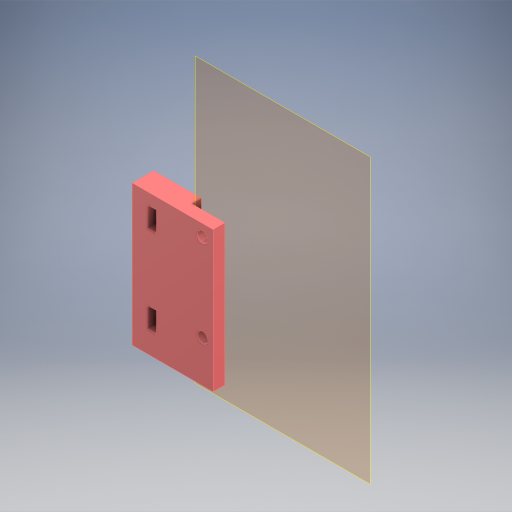
# Autodesk Inventor part: foot_right_connection
Saved by Autodesk Inventor 2024 (Build 280153000, 153)
## iProperties
Created: 2024-09-03
Part Number: foot_right_connection
Material: PMMA 플라스틱
Document SubType Name: Modeling
Designer: msi
Density: 1.188 g/cm^3
Appearance: 매끄러움 - 빨간색
Author: msi
Autodesk Inventor part; units mm, degrees
ref_plane "YZ Plane" through (0, 0, 0) normal (1, 0, 0) x (0, 1, 0)
ref_plane "XZ Plane" through (0, 0, 0) normal (0, 1, 0) x (-1, 0, 0)
ref_plane "XY Plane" through (0, 0, 0) normal (0, 0, 1) x (1, 0, 0)
ref_plane "작업 평면1" through (0, 0, 0) normal (0, 0, 1) x (1, 0, 0)
sketch "스케치2" plane through (0, 0, 0) normal (0, 0, 1) x (1, 0, 0)
  line L0 (13.5, -39.75) -> (11.5, -39.75) projected
  arc A0 (11.5, -39.75) -> (9.25, -42) centre (11.5, -42) ccw projected
  line L1 (9.25, -42) -> (9.25, -44) projected
  arc A1 (8.25, -45) -> (9.25, -44) centre (8.25, -44) ccw projected
  line L2 (8.25, -45) -> (-8.25, -45) projected
  arc A2 (-9.25, -44) -> (-8.25, -45) centre (-8.25, -44) ccw projected
  line L3 (-9.25, -44) -> (-9.25, -42) projected
  arc A3 (-9.25, -42) -> (-11.5, -39.75) centre (-11.5, -42) ccw projected
  line L4 (-11.5, -39.75) -> (-13.5, -39.75) projected
  arc A4 (-14.5, -38.75) -> (-13.5, -39.75) centre (-13.5, -38.75) ccw projected
  line L5 (-14.5, -38.75) -> (-14.5, 8.25) projected
  arc A5 (-13.5, 9.25) -> (-14.5, 8.25) centre (-13.5, 8.25) ccw projected
  line L6 (-13.5, 9.25) -> (-11.5, 9.25) projected
  arc A6 (-11.5, 9.25) -> (-9.25, 11.5) centre (-11.5, 11.5) ccw projected
  line L7 (-9.25, 11.5) -> (-9.25, 14.5) projected
  line L8 (-15, 14.5) -> (-9.25, 14.5) projected
  line L9 (-20.1, 8.5) -> (-15, 14.5) projected
  line L10 (-20.1, -44.6) -> (-20.1, 8.5) projected
  line L11 (-15, -50.6) -> (-20.1, -44.6) projected
  line L12 (15, -50.6) -> (-15, -50.6) projected
  line L13 (20.1, -44.6) -> (15, -50.6) projected
  line L14 (20.1, 8.5) -> (20.1, -44.6) projected
  line L15 (15, 14.5) -> (20.1, 8.5) projected
  line L16 (9.25, 14.5) -> (15, 14.5) projected
  line L17 (9.25, 14.5) -> (9.25, 11.5) projected
  arc A7 (9.25, 11.5) -> (11.5, 9.25) centre (11.5, 11.5) ccw projected
  line L18 (11.5, 9.25) -> (13.5, 9.25) projected
  arc A8 (14.5, 8.25) -> (13.5, 9.25) centre (13.5, 8.25) ccw projected
  line L19 (14.5, 8.25) -> (14.5, -38.75) projected
  arc A9 (13.5, -39.75) -> (14.5, -38.75) centre (13.5, -38.75) ccw projected
  circle A10 centre (17.3, 4) radius 1.35 projected
  circle A11 centre (17.3, -18) radius 1.35 projected
  circle A12 centre (11, -47.8) radius 1.35 projected
  circle A13 centre (-17.3, 4) radius 1.35 projected
  circle A14 centre (-17.3, -18) radius 1.35 projected
  circle A15 centre (-11, -47.8) radius 1.35 projected
  circle A16 centre (17.3, -40) radius 1.35 projected
  circle A17 centre (-17.3, -40) radius 1.35 projected
  line L20 (-43, 2.0766) -> (-43, -42.1766) projected
  line L21 (-14.6, 8.25) -> (-14.6, -38.75)
  arc A18 (-14.6, -38.75) -> (-13.5, -39.85) centre (-13.5, -38.75) ccw
  line L22 (-13.5, -39.85) -> (-11.5, -39.85)
  arc A19 (-9.35, -42) -> (-11.5, -39.85) centre (-11.5, -42) ccw
  line L23 (-9.35, -42) -> (-9.35, -44)
  arc A20 (-9.35, -44) -> (-8.25, -45.1) centre (-8.25, -44) ccw
  line L24 (-8.25, -45.1) -> (8.25, -45.1)
  arc A21 (8.25, -45.1) -> (9.35, -44) centre (8.25, -44) ccw
  line L25 (9.35, -44) -> (9.35, -42)
  arc A22 (11.5, -39.85) -> (9.35, -42) centre (11.5, -42) ccw
  line L26 (11.5, -39.85) -> (13.5, -39.85)
  arc A23 (13.5, -39.85) -> (14.6, -38.75) centre (13.5, -38.75) ccw
  line L27 (14.6, -38.75) -> (14.6, 8.25)
  arc A24 (14.6, 8.25) -> (13.5, 9.35) centre (13.5, 8.25) ccw
  line L28 (13.5, 9.35) -> (11.5, 9.35)
  arc A25 (9.35, 11.5) -> (11.5, 9.35) centre (11.5, 11.5) ccw
  line L29 (9.35, 11.5) -> (9.35, 14.4)
  line L30 (9.35, 14.4) -> (14.9538, 14.4)
  line L31 (14.9538, 14.4) -> (20, 8.4632)
  line L32 (20, 8.4632) -> (20, -44.5632)
  line L33 (20, -44.5632) -> (14.9538, -50.5)
  line L34 (14.9538, -50.5) -> (-14.9538, -50.5)
  line L35 (-20, -15) -> (-20, 8.4632)
  line L36 (-20, 8.4632) -> (-14.9538, 14.4)
  line L37 (-14.9538, 14.4) -> (-9.35, 14.4)
  line L38 (-9.35, 14.4) -> (-9.35, 11.5)
  arc A26 (-11.5, 9.35) -> (-9.35, 11.5) centre (-11.5, 11.5) ccw
  line L39 (-11.5, 9.35) -> (-13.5, 9.35)
  arc A27 (-13.5, 9.35) -> (-14.6, 8.25) centre (-13.5, 8.25) ccw
  line L40 (-20, -15) -> (-14.6, -15)
  line L41 (-14.6, -15) -> (-14.6, -45)
  line L42 (-43, -15) -> (-20, -15)
  line L43 (-35, -45) -> (-35, -50.5)
  line L44 (-35, -50.5) -> (-14.6, -50.5)
  line L45 (-14.6, -50.5) -> (-14.6, -45)
  line L46 (-35, -45) -> (-35, -15)
  point P0 (0, 0)
  point P1 (-14.6, -38.75)
  point P2 (-14.6, -50.5)
  point P3 (-14.6, -38.75)
  dimension "d1" = 0.1
  dimension "d27" = 20.4
  constraints: 52 end point, 20 point on circle, 10 centre point, 2 point on line, 1 parallel, 1 perpendicular, 26 other
  measures "d1" distance between parallel lines of L5 L21
  measures "d27" distance between parallel lines of L43 L45
extrude "돌출8" add sketch "스케치2" along normal blind 3 contours L44 L43 L46 L42 L10 L11 | L11 L10 L42 L40 L21 L41 L45 L34 L44
sketch "스케치10" plane through (-35, -50.5, 0) normal (-1, 0, 0) x (0, 0, 1)
  arc A0 (-36.5808, 54.2636) -> (-37.1, 52.5766) centre (-34.1, 52.5766) ccw projected
  line L0 (-37.1, 8.3234) -> (-37.1, 52.5766) projected
  arc A1 (-37.1, 8.3234) -> (-36.5808, 6.6364) centre (-34.1, 8.3234) ccw projected
  line L1 (-32.8929, 1.2131) -> (-36.5808, 6.6364) projected
  arc A2 (-32.8929, 1.2131) -> (-30.4121, -0.1) centre (-30.4121, 2.9) ccw projected
  line L2 (-3.5879, -0.1) -> (-30.4121, -0.1) projected
  arc A3 (-3.5879, -0.1) -> (-1.1071, 1.2131) centre (-3.5879, 2.9) ccw projected
  line L3 (2.5808, 6.6364) -> (-1.1071, 1.2131) projected
  arc A4 (2.5808, 6.6364) -> (3.1, 8.3234) centre (0.1, 8.3234) ccw projected
  line L4 (3.1, 52.5766) -> (3.1, 8.3234) projected
  arc A5 (3.1, 52.5766) -> (2.5808, 54.2636) centre (0.1, 52.5766) ccw projected
  line L5 (-1.4047, 60.1246) -> (2.5808, 54.2636) projected
  arc A6 (-1.4047, 60.1246) -> (-3.0586, 61) centre (-3.0586, 59) ccw projected
  line L6 (-9.35, 61) -> (-3.0586, 61) projected
  arc A7 (-7.85, 59.5) -> (-9.35, 61) centre (-9.35, 59.5) ccw projected
  line L7 (-7.85, 59.5) -> (-7.85, 58) projected
  arc A8 (-7.85, 58) -> (-5.5, 55.65) centre (-5.5, 58) ccw projected
  line L8 (-5.5, 55.65) -> (-3.5, 55.65) projected
  arc A9 (-2.5, 54.65) -> (-3.5, 55.65) centre (-3.5, 54.65) ccw projected
  line L9 (-2.5, 54.65) -> (-2.5, 11.85) projected
  arc A10 (-3.5, 10.85) -> (-2.5, 11.85) centre (-3.5, 11.85) ccw projected
  line L10 (-3.5, 10.85) -> (-5.5, 10.85) projected
  arc A11 (-5.5, 10.85) -> (-7.85, 8.5) centre (-5.5, 8.5) ccw projected
  line L11 (-7.85, 8.5) -> (-7.85, 6.5) projected
  arc A12 (-8.85, 5.5) -> (-7.85, 6.5) centre (-8.85, 6.5) ccw projected
  line L12 (-8.85, 5.5) -> (-25.15, 5.5) projected
  arc A13 (-26.15, 6.5) -> (-25.15, 5.5) centre (-25.15, 6.5) ccw projected
  line L13 (-26.15, 6.5) -> (-26.15, 8.5) projected
  arc A14 (-26.15, 8.5) -> (-28.5, 10.85) centre (-28.5, 8.5) ccw projected
  line L14 (-28.5, 10.85) -> (-30.5, 10.85) projected
  arc A15 (-31.5, 11.85) -> (-30.5, 10.85) centre (-30.5, 11.85) ccw projected
  line L15 (-31.5, 11.85) -> (-31.5, 54.65) projected
  arc A16 (-30.5, 55.65) -> (-31.5, 54.65) centre (-30.5, 54.65) ccw projected
  line L16 (-30.5, 55.65) -> (-28.5, 55.65) projected
  arc A17 (-28.5, 55.65) -> (-26.15, 58) centre (-28.5, 58) ccw projected
  line L17 (-26.15, 58) -> (-26.15, 59.5) projected
  arc A18 (-24.65, 61) -> (-26.15, 59.5) centre (-24.65, 59.5) ccw projected
  line L18 (-30.9414, 61) -> (-24.65, 61) projected
  arc A19 (-30.9414, 61) -> (-32.5953, 60.1246) centre (-30.9414, 59) ccw projected
  line L19 (-36.5808, 54.2636) -> (-32.5953, 60.1246) projected
  circle A20 centre (0.3, 52) radius 1.35 projected
  circle A21 centre (0.3, 30) radius 1.35 projected
  circle A22 centre (-6, 2.7) radius 1.35 projected
  circle A23 centre (-34.3, 52) radius 1.35 projected
  circle A24 centre (-34.3, 30) radius 1.35 projected
  circle A25 centre (-28, 2.7) radius 1.35 projected
  circle A26 centre (0.3, 8) radius 1.35 projected
  circle A27 centre (-34.3, 8) radius 1.35 projected
  line L20 (0, 35.5) -> (0, 0) projected
  line L21 (0, 0) -> (3, 0) projected
  line L22 (3, 35.5) -> (3, 0) projected
  line L23 (0, 35.5) -> (3, 35.5) projected
  line L24 (-2.4, 11.85) -> (-2.4, 54.65)
  arc A28 (-2.4, 54.65) -> (-3.5, 55.75) centre (-3.5, 54.65) ccw
  line L25 (-3.5, 55.75) -> (-5.5, 55.75)
  arc A29 (-7.75, 58) -> (-5.5, 55.75) centre (-5.5, 58) ccw
  line L26 (-7.75, 58) -> (-7.75, 59.5)
  arc A30 (-7.75, 59.5) -> (-10.1246, 60.9) centre (-9.35, 59.5) ccw
  line L27 (-10.1246, 60.9) -> (-3.0586, 60.9)
  arc A31 (-1.4874, 60.0684) -> (-3.0586, 60.9) centre (-3.0586, 59) ccw
  line L28 (-1.4874, 60.0684) -> (2.4981, 54.2073)
  arc A32 (3, 52.5766) -> (2.4981, 54.2073) centre (0.1, 52.5766) ccw
  line L29 (3, 52.5766) -> (3, 8.3234)
  arc A33 (2.4981, 6.6927) -> (3, 8.3234) centre (0.1, 8.3234) ccw
  line L30 (2.4981, 6.6927) -> (0, 3.019)
  arc A34 (-3.5879, 0) -> (-2.4, 0.2545) centre (-3.5879, 2.9) ccw
  line L31 (-3.5879, 0) -> (-30.4121, 0)
  arc A35 (-32.8102, 1.2693) -> (-30.4121, 0) centre (-30.4121, 2.9) ccw
  line L32 (-32.8102, 1.2693) -> (-36.4981, 6.6927)
  arc A36 (-37, 8.3234) -> (-36.4981, 6.6927) centre (-34.1, 8.3234) ccw
  line L33 (-37, 8.3234) -> (-37, 52.5766)
  arc A37 (-36.4981, 54.2073) -> (-37, 52.5766) centre (-34.1, 52.5766) ccw
  line L34 (-36.4981, 54.2073) -> (-32.5126, 60.0684)
  arc A38 (-30.9414, 60.9) -> (-32.5126, 60.0684) centre (-30.9414, 59) ccw
  line L35 (-30.9414, 60.9) -> (-25.4246, 60.9)
  arc A39 (-25.4246, 60.9) -> (-26.25, 59.5) centre (-24.65, 59.5) ccw
  line L36 (-26.25, 59.5) -> (-26.25, 58)
  arc A40 (-28.5, 55.75) -> (-26.25, 58) centre (-28.5, 58) ccw
  line L37 (-28.5, 55.75) -> (-30.5, 55.75)
  arc A41 (-30.5, 55.75) -> (-31.6, 54.65) centre (-30.5, 54.65) ccw
  line L38 (-31.6, 54.65) -> (-31.6, 11.85)
  arc A42 (-31.6, 11.85) -> (-30.5, 10.75) centre (-30.5, 11.85) ccw
  line L39 (-30.5, 10.75) -> (-28.5, 10.75)
  arc A43 (-26.25, 8.5) -> (-28.5, 10.75) centre (-28.5, 8.5) ccw
  line L40 (-26.25, 8.5) -> (-26.25, 6.5)
  arc A44 (-26.25, 6.5) -> (-25.15, 5.4) centre (-25.15, 6.5) ccw
  line L41 (-25.15, 5.4) -> (-8.85, 5.4)
  arc A45 (-8.85, 5.4) -> (-7.75, 6.5) centre (-8.85, 6.5) ccw
  line L42 (-7.75, 6.5) -> (-7.75, 8.5)
  arc A46 (-5.5, 10.75) -> (-7.75, 8.5) centre (-5.5, 8.5) ccw
  line L43 (-5.5, 10.75) -> (-3.5, 10.75)
  arc A47 (-3.5, 10.75) -> (-2.4, 11.85) centre (-3.5, 11.85) ccw
  line L44 (0, 0) -> (-2.4, 0)
  line L45 (-2.4, 0) -> (-2.4, 35.5)
  line L46 (-2.4, 35.5) -> (0, 35.5)
  line L47 (0, 35.5) -> (0, 0)
  point P0 (0, 50.5)
  point P1 (0, 6.6838)
  point P2 (0, 9.3162)
  point P3 (0, 28.6838)
  point P4 (0, 31.3162)
  point P5 (0, 35.5)
  point P6 (-2.4, 11.85)
  dimension "d30" = 0.1
  constraints: 48 end point, 40 point on circle, 20 centre point, 3 point on line, 2 parallel, 1 horizontal, 1 perpendicular, 36 other
  measures "d30" distance between parallel lines of L9 L24
extrude "돌출10" add sketch "스케치10" against normal blind 12 contours L45 L24 L46 L20 A21 A26 L3 A3 | A3 L3 L20 L44 L45
sketch "스케치12" plane through (-35, -50.5, 3) normal (-1, 0, 0) x (0, 0, 1)
  line L0 (-5.5579, 8) -> (-4.1289, 5.525) projected
  arc A0 (-39.5808, 54.2636) -> (-40.1, 52.5766) centre (-37.1, 52.5766) ccw projected
  line L1 (-40.1, 8.3234) -> (-40.1, 52.5766) projected
  arc A1 (-40.1, 8.3234) -> (-39.5808, 6.6364) centre (-37.1, 8.3234) ccw projected
  line L2 (-35.8929, 1.2131) -> (-39.5808, 6.6364) projected
  arc A2 (-35.8929, 1.2131) -> (-33.4121, -0.1) centre (-33.4121, 2.9) ccw projected
  line L3 (-6.5879, -0.1) -> (-33.4121, -0.1) projected
  arc A3 (-6.5879, -0.1) -> (-4.1071, 1.2131) centre (-6.5879, 2.9) ccw projected
  line L4 (-0.4192, 6.6364) -> (-4.1071, 1.2131) projected
  arc A4 (-0.4192, 6.6364) -> (0.1, 8.3234) centre (-2.9, 8.3234) ccw projected
  line L5 (0.1, 52.5766) -> (0.1, 8.3234) projected
  arc A5 (0.1, 52.5766) -> (-0.4192, 54.2636) centre (-2.9, 52.5766) ccw projected
  line L6 (-4.4047, 60.1246) -> (-0.4192, 54.2636) projected
  arc A6 (-4.4047, 60.1246) -> (-6.0586, 61) centre (-6.0586, 59) ccw projected
  line L7 (-12.35, 61) -> (-6.0586, 61) projected
  arc A7 (-10.85, 59.5) -> (-12.35, 61) centre (-12.35, 59.5) ccw projected
  line L8 (-10.85, 59.5) -> (-10.85, 58) projected
  arc A8 (-10.85, 58) -> (-8.5, 55.65) centre (-8.5, 58) ccw projected
  line L9 (-8.5, 55.65) -> (-6.5, 55.65) projected
  arc A9 (-5.5, 54.65) -> (-6.5, 55.65) centre (-6.5, 54.65) ccw projected
  line L10 (-5.5, 54.65) -> (-5.5, 11.85) projected
  arc A10 (-6.5, 10.85) -> (-5.5, 11.85) centre (-6.5, 11.85) ccw projected
  line L11 (-6.5, 10.85) -> (-8.5, 10.85) projected
  arc A11 (-8.5, 10.85) -> (-10.85, 8.5) centre (-8.5, 8.5) ccw projected
  line L12 (-10.85, 8.5) -> (-10.85, 6.5) projected
  arc A12 (-11.85, 5.5) -> (-10.85, 6.5) centre (-11.85, 6.5) ccw projected
  line L13 (-11.85, 5.5) -> (-28.15, 5.5) projected
  arc A13 (-29.15, 6.5) -> (-28.15, 5.5) centre (-28.15, 6.5) ccw projected
  line L14 (-29.15, 6.5) -> (-29.15, 8.5) projected
  arc A14 (-29.15, 8.5) -> (-31.5, 10.85) centre (-31.5, 8.5) ccw projected
  line L15 (-31.5, 10.85) -> (-33.5, 10.85) projected
  arc A15 (-34.5, 11.85) -> (-33.5, 10.85) centre (-33.5, 11.85) ccw projected
  line L16 (-34.5, 11.85) -> (-34.5, 54.65) projected
  arc A16 (-33.5, 55.65) -> (-34.5, 54.65) centre (-33.5, 54.65) ccw projected
  line L17 (-33.5, 55.65) -> (-31.5, 55.65) projected
  arc A17 (-31.5, 55.65) -> (-29.15, 58) centre (-31.5, 58) ccw projected
  line L18 (-29.15, 58) -> (-29.15, 59.5) projected
  arc A18 (-27.65, 61) -> (-29.15, 59.5) centre (-27.65, 59.5) ccw projected
  line L19 (-33.9414, 61) -> (-27.65, 61) projected
  arc A19 (-33.9414, 61) -> (-35.5953, 60.1246) centre (-33.9414, 59) ccw projected
  line L20 (-39.5808, 54.2636) -> (-35.5953, 60.1246) projected
  circle A20 centre (-2.7, 52) radius 1.35 projected
  circle A21 centre (-2.7, 30) radius 1.35 projected
  circle A22 centre (-9, 2.7) radius 1.35 projected
  circle A23 centre (-37.3, 52) radius 1.35 projected
  circle A24 centre (-37.3, 30) radius 1.35 projected
  circle A25 centre (-31, 2.7) radius 1.35 projected
  circle A26 centre (-2.7, 8) radius 1.35 projected
  circle A27 centre (-37.3, 8) radius 1.35 projected
  circle A28 centre (-2.7, 8) radius 1.35
  circle A29 centre (-2.7, 30) radius 1.35
  point P0 (-3, 50.5)
  dimension "d35" = 2.7
  dimension "d36" = 2.7
  constraints: 2 centre point, 2 coincident
  measures "d35" diameter of A28
  measures "d36" diameter of A29
extrude "돌출11" cut sketch "스케치12" against normal blind 10 contours A21 | A26
sketch "스케치13" plane through (0, 0, 3) normal (0, 0, 1) x (1, 0, 0)
  line L0 (-25, -43.85) -> (-35, -43.85) projected
  line L1 (-25, -41.15) -> (-35, -41.15) projected
  line L2 (-25, -21.85) -> (-35, -21.85) projected
  line L3 (-25, -19.15) -> (-35, -19.15) projected
  line L4 (-30, -43.85) -> (-30, -41.15)
  line L5 (-30, -19.15) -> (-30, -21.85)
  line L6 (-28.9, -39.9) -> (-31.1, -39.9)
  line L7 (-31.1, -39.9) -> (-31.1, -45.1)
  line L8 (-31.1, -45.1) -> (-28.9, -45.1)
  line L9 (-28.9, -45.1) -> (-28.9, -39.9)
  line L10 (-28.9, -39.9) -> (-31.1, -45.1) construction
  line L11 (-31.1, -39.9) -> (-28.9, -45.1) construction
  line L12 (-28.9, -17.9) -> (-31.1, -17.9)
  line L13 (-31.1, -17.9) -> (-31.1, -23.1)
  line L14 (-31.1, -23.1) -> (-28.9, -23.1)
  line L15 (-28.9, -23.1) -> (-28.9, -17.9)
  line L16 (-28.9, -17.9) -> (-31.1, -23.1) construction
  line L17 (-31.1, -17.9) -> (-28.9, -23.1) construction
  point P0 (0, 0)
  point P1 (-30, -42.5)
  point P2 (-30, -20.5)
  dimension "d39" = 2.2
  dimension "d40" = 5.2
  dimension "d41" = 2.2
  dimension "d42" = 5.2
  constraints: 28 end point, 10 midpoint, 4 parallel, 2 horizontal, 2 perpendicular
  measures "d39" distance of L8.end L7.end
  measures "d40" distance of L7.end L6.end
  measures "d41" distance of L14.end L13.end
  measures "d42" distance of L13.end L12.end
extrude "돌출12" cut sketch "스케치13" against normal blind 10
